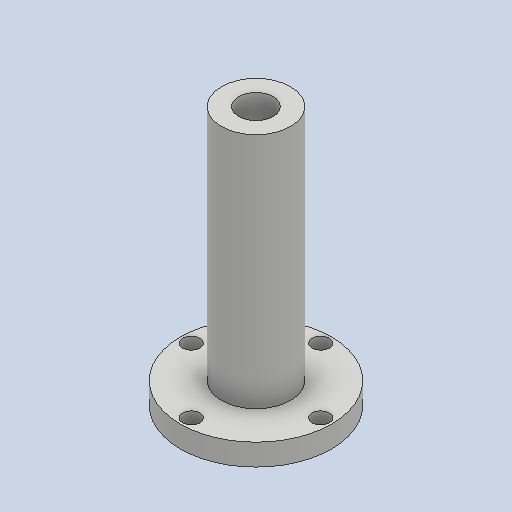
# Autodesk Inventor part: VerticalBearing
Saved by Autodesk Inventor 2023 (Build 270158000, 158)
## iProperties
Created: 2022-08-28
Part Number: VerticalBearing
Material: Generic
Document SubType Name: Modeling
Designer: Nathann
Density: 1 g/cm^3
Appearance: Default
Author: Nathann
Autodesk Inventor part; units mm, degrees
ref_plane "YZ Plane" through (0, 0, 0) normal (1, 0, 0) x (0, 1, 0)
ref_plane "XZ Plane" through (0, 0, 0) normal (0, 1, 0) x (-1, 0, 0)
ref_plane "XY Plane" through (0, 0, 0) normal (0, 0, 1) x (1, 0, 0)
sketch "Sketch3" plane through (0, 0, 0) normal (0, 0, 1) x (1, 0, 0)
  circle A0 centre (0, 0) radius 4
  circle A1 centre (0, 0) radius 17.5
  dimension "d0" = 8
  dimension "d1" = 35
  constraints: 2 centre point, 2 coincident
  measures "d0" diameter of A0
  measures "d1" diameter of A1
extrude "Extrusion1" add sketch "Sketch3" along normal blind 5
sketch "Sketch4" plane through (0, 0, 5) normal (0, 0, 1) x (1, 0, 0)
  circle A0 centre (0, 0) radius 4
  circle A1 centre (0, 0) radius 8
  dimension "d4" = 16
  dimension "d5" = 8
  constraints: 2 centre point, 2 coincident
  measures "d4" diameter of A1
  measures "d5" diameter of A0
extrude "Extrusion2" add sketch "Sketch4" along normal blind 55
sketch "Sketch5" plane through (0, 0, 0) normal (0, 0, -1) x (-1, 0, 0)
  circle A0 centre (15, 0) radius 2
  circle A1 centre (0, 15) radius 2
  circle A2 centre (0, -15) radius 2
  circle A3 centre (-15, 0) radius 2
  point P0 (0, 0)
  dimension "d8" = 4
  dimension "d9" = 15
  dimension "d10" = 15
  dimension "d11" = 15
  dimension "d12" = 15
  dimension "d13" = 4
  dimension "d14" = 4
  dimension "d15" = 4
  constraints: 4 centre point
  measures "d8" diameter of A3
  measures "d9" distance of point (0, 0) A1.centre
  measures "d10" distance of point (0, 0) A2.centre
  measures "d11" distance of point (0, 0) A3.centre
  measures "d12" distance of point (0, 0) A0.centre
  measures "d13" diameter of A2
  measures "d14" diameter of A0
  measures "d15" diameter of A1
extrude "Extrusion3" cut sketch "Sketch5" against normal through all
equation "\"d0\" = RodDiameter"
equation "\"d4\" = VerticalBearingOD"
equation "\"d5\" = RodDiameter"
equation "\"d9\" = 0.5 * VerticalBearingMountingHoleDiameter"
equation "\"d10\" = 0.5 * VerticalBearingMountingHoleDiameter"
equation "\"d11\" = 0.5 * VerticalBearingMountingHoleDiameter"
equation "\"d12\" = 0.5 * VerticalBearingMountingHoleDiameter"
equation "\"d13\" = d8"
equation "\"d14\" = d8"
equation "\"d15\" = d8"
equation "\"RodDiameter\" = 8"
equation "\"VerticalBearingOD\" = 16"
equation "\"PrintingClearance\" = 0.2"
equation "\"TubeID\" = 18"
equation "\"VerticalBearingMountingHoleDiameter\" = 30"
body "Solid1"
